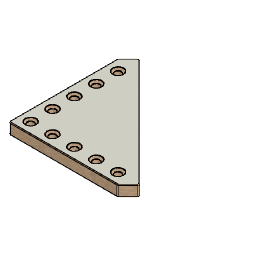
model (Autodesk Fusion 360 design; units mm, degrees)
Autodesk Fusion 360 part; units mm, degrees
sketch "Sketch1" plane through (0, 0, 0) normal (0, 0, 1) x (1, 0, 0) in component "square"
  line L0 (0, 160) -> (0, 0)
  line L1 (0, 0) -> (160, 0)
  line L2 (160, 0) -> (160, 32)
  line L3 (160, 32) -> (32, 32)
  line L4 (32, 32) -> (32, 160)
  line L5 (32, 160) -> (0, 160)
  line L6 (0, 0) -> (32, 32) construction
  line L7 (32, 160) -> (160, 32) construction
  line L8 (32, 32) -> (96, 96) construction
  circle A0 centre (16, 16) radius 4.7625
  line L9 (16, 16) -> (0, 16) construction
  line L10 (16, 16) -> (32, 16) construction
  circle A1 centre (16, 48) radius 4.7625
  circle A2 centre (16, 80) radius 4.7625
  circle A3 centre (16, 112) radius 4.7625
  circle A4 centre (16, 144) radius 4.7625
  line L11 (16, 16) -> (16, 0) construction
  circle A5 centre (48, 16) radius 4.7625
  circle A6 centre (80, 16) radius 4.7625
  circle A7 centre (112, 16) radius 4.7625
  circle A8 centre (144, 16) radius 4.7625
  line L12 (30.8775, 44.3479) -> (37.6127, 37.6127) construction
  line L13 (37.6127, 37.6127) -> (44.3479, 30.8775) construction
  circle A9 centre (37.6127, 37.6127) radius 9.525
  dimension "d6" = 32
  dimension "d7" = 160
  dimension "d8" = 9.525
  dimension "d12" = 0
  dimension "d13" = 128
  dimension "d16" = 128
  dimension "d17" = 0
  dimension "d22" = 32
  dimension "d33" = 19.05
  dimension "d34" = 7.9375
  constraint coincident L0.end L1.start
  constraint vertical L0
  constraint horizontal L5
  constraint vertical L4
  constraint vertical L2
  constraint horizontal L1
  constraint horizontal L3
  constraint perpendicular L6 L7
  constraint coincident L7 L8.end
  constraint collinear L6 L8
  constraint midpoint L7 L8.end
  constraint coincident A0.centre L9.start
  constraint coincident L0 L9.end
  constraint perpendicular L0 L9
  constraint coincident L4 L10.end
  constraint perpendicular L4 L10
  constraint equal L9 L10
  constraint coincident L1 L11.end
  constraint perpendicular L1 L11
  constraint equal L10 L11
  constraint coincident L8 L12.end
  constraint perpendicular L8 L12
  constraint collinear L12 L13
  constraint equal L12 L13
  constraint coincident L12.end L13.start
  constraint coincident L12.start A9
  measures "d6" distance of L0.start L4.end
  measures "d7" distance of L0.start L0.end
  measures "d8" diameter of A0
  measures "d22" distance of A3.centre A4.centre
  measures "d33" diameter of A9
  measures "d34" distance of L3.end L12.end
extrude "Extrude1" add sketch "Sketch1" along normal blind 16.3 contours L0 L1 L2 L3 L4 L5 A9 makes body 1 in component "square"
chamfer "Chamfer1" distance 3 angle 45 9 faces at (20.7566, 15.7626, 10.8667) (52.7566, 15.7626, 10.8667) (84.7566, 15.7626, 10.8667) (116.7566, 15.7626, 10.8667) (143.8813, 20.761, 10.8667) (20.7566, 47.7626, 10.8667) (11.8175, 77.7223, 10.8667) (20.6681, 111.0563, 10.8667) (11.3848, 142.8248, 10.8667) on bodies 1 in component "square"
fillet "Fillet2" radius 5 5 edges at (0, 160, 8.15) (0, 0, 8.15) (160, 0, 8.15) (160, 32, 8.15) (32, 160, 8.15) on bodies 1 in component "square"
fillet "Fillet2" radius 5 2 edges at (32, 45.3084, 8.15) (45.3084, 32, 8.15) on bodies 1 in component "square"
fillet "Fillet1" radius 1 2 faces at (79.8066, 2.7531, 16.3) (79.8066, 2.7531, 0) on bodies 1 in component "square"
fillet "Fillet1" radius 1 9 faces at (11.9362, 77.5167, 9.8667) (20.6681, 111.0563, 9.8667) (11.3319, 143.0563, 9.8667) (20.7566, 47.7626, 9.8667) (20.7566, 15.7626, 9.8667) (52.7566, 15.7626, 9.8667) (84.7566, 15.7626, 9.8667) (116.7566, 15.7626, 9.8667) (144.1187, 20.761, 9.8667) on bodies 1 in component "square"
sketch "Sketch1 (2)" plane through (0, 0, 0) normal (0, 0, 1) x (1, 0, 0) in component "triangle"
  line L0 (0, 0) -> (0, 160)
  line L1 (160, 0) -> (0, 0)
  line L2 (0, 160) -> (16.2635, 176.2635)
  line L3 (16.2635, 176.2635) -> (176.2635, 16.2635)
  line L4 (176.2635, 16.2635) -> (160, 0)
  circle A0 centre (16.2635, 16.2635) radius 4.7625
  line L5 (16.2635, 16.2635) -> (0, 16.2635) construction
  line L6 (16.2635, 16.2635) -> (16.2635, 0) construction
  line L7 (16.2635, 16.2635) -> (16.2635, 176.2635) construction
  circle A1 centre (16.2635, 48.2635) radius 4.7625
  circle A2 centre (16.2635, 80.2635) radius 4.7625
  circle A3 centre (16.2635, 112.2635) radius 4.7625
  circle A4 centre (16.2635, 144.2635) radius 4.7625
  circle A5 centre (48.2635, 16.2635) radius 4.7625
  circle A6 centre (80.2635, 16.2635) radius 4.7625
  circle A7 centre (112.2635, 16.2635) radius 4.7625
  circle A8 centre (144.2635, 16.2635) radius 4.7625
  line L8 (160, 0) -> (192.5269, 0) construction
  line L9 (192.5269, 0) -> (176.2635, 16.2635) construction
  dimension "d44" = 9.525
  dimension "d50" = 0
  dimension "d51" = 32
  dimension "d55" = 32
  dimension "d56" = 0
  dimension "d58" = 16.2635
  dimension "d67" = 192.5269
  dimension "d68" = 48.2635
  dimension "d69" = 144.2635
  dimension "d70" = 112.2635
  dimension "d71" = 80.2635
  dimension "d73" = 160
  dimension "d74" = 23
  constraint coincident L0.start L1.end
  constraint vertical L0
  constraint perpendicular L0 L1
  constraint perpendicular L2 L3
  constraint perpendicular L3 L4
  constraint equal L2 L4
  constraint coincident A0.centre L5.start
  constraint coincident L0 L5.end
  constraint perpendicular L0 L5
  constraint coincident L1 L6.end
  constraint perpendicular L1 L6
  constraint equal L5 L6
  constraint collinear L6 L7
  constraint equal L0 L1
  constraint horizontal L8
  constraint perpendicular L4 L9
  measures "d44" diameter of A0
  measures "d58" distance of L0 A0.centre
  measures "d67" distance of L0.start L8.end
  measures "d68" distance of L0 A5.centre
  measures "d69" distance of L0 A8.centre
  measures "d70" distance of L0 A7.centre
  measures "d71" distance of L0 A6.centre
  measures "d73" distance of L1.start L0.start
  measures "d74" distance of L3.end L8.end
extrude "Extrude1'" add sketch "Sketch1 (2)" along normal blind 16.3 separate body makes body 2 in component "triangle"
chamfer "Chamfer1'" distance 3 angle 45 9 faces at (11.6482, 143.0883, 10.8667) (12.0809, 109.9858, 10.8667) (12.0809, 77.9858, 10.8667) (21.02, 48.0261, 10.8667) (21.02, 16.0261, 10.8667) (53.02, 16.0261, 10.8667) (85.02, 16.0261, 10.8667) (117.02, 16.0261, 10.8667) (144.1447, 21.0245, 10.8667) on bodies 2 in component "triangle"
fillet "Fillet1'" radius 3 5 edges at (0, 0, 8.15) (160, 0, 8.15) (176.2635, 16.2635, 8.15) (16.2635, 176.2635, 8.15) (0, 160, 8.15) on bodies 2 in component "triangle"
fillet "Fillet2'" radius 1 11 faces at (63.854, 93.5104, 16.3) (63.854, 93.5104, 0) (21.02, 48.0261, 9.8667) (12.1997, 77.7801, 9.8667) (12.1997, 109.7801, 9.8667) (11.5954, 143.3198, 9.8667) (21.02, 16.0261, 9.8667) (53.02, 16.0261, 9.8667) (85.02, 16.0261, 9.8667) (117.02, 16.0261, 9.8667) (144.3822, 21.0245, 9.8667) on bodies 2 in component "triangle"
component "square" placed x (1, 0, 0) y (0, 1, 0) z (0, 0, 1) at (0, 0, 0)
component "triangle" placed x (1, 0, 0) y (0, 1, 0) z (0, 0, 1) at (0, 0, 0)
equation "squareWidth = 32 mm"
equation "referenceSurfaceLength = 160 mm"
equation "materialThickness = 16.3 mm"
equation "clampDiameter = 8 mm"
equation "clampHoleDiameter = 3 / 8 * 1\""
equation "d6 = squareWidth"
equation "d7 = referenceSurfaceLength"
equation "d8 = clampHoleDiameter"
equation "squareHoleCount = 5"
equation "d11 = squareHoleCount"
equation "d13 = referenceSurfaceLength - squareWidth"
equation "d14 = squareHoleCount"
equation "d16 = referenceSurfaceLength - squareWidth"
equation "d23 = materialThickness"
equation "chamferSize = 3 mm"
equation "d26 = chamferSize"
equation "reliefDiameter = 3 / 4 * 1 in"
equation "reliefDepth = reliefDiameter / 2 / 6"
equation "d33 = reliefDiameter"
equation "d34 = reliefDiameter / 2 - reliefDepth"
equation "roundingRadius = 5 mm"
equation "d39 = roundingRadius"
equation "d41 = roundingRadius"
equation "d44 = clampHoleDiameter"
equation "triangleCutDepth = 23 mm"
equation "d49 = squareHoleCount"
equation "triangleHoleSpacing = 32 mm"
equation "d53 = squareHoleCount"
equation "d55 = triangleHoleSpacing"
equation "d59 = materialThickness"
equation "d61 = chamferSize"
equation "d63 = chamferSize"
equation "d73 = referenceSurfaceLength"
equation "d74 = triangleCutDepth"
